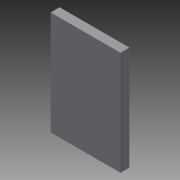
# Autodesk Inventor part: anker20Ah
Saved by Autodesk Inventor 2015 (Build 190159000, 159)
## iProperties
Created: 2014-09-23
Part Number: anker20Ah
Material: Generic
Document SubType Name: Modeling
Designer: ericd_000
Density: 1 g/cm^3
Appearance: Default
Author: ericd_000
Autodesk Inventor part; units mm, degrees
ref_plane "YZ Plane" through (0, 0, 0) normal (1, 0, 0) x (0, 1, 0)
ref_plane "XZ Plane" through (0, 0, 0) normal (0, 1, 0) x (-1, 0, 0)
ref_plane "XY Plane" through (0, 0, 0) normal (0, 0, 1) x (1, 0, 0)
sketch "Sketch1" plane through (0, 0, 0) normal (0, 1, 0) x (-1, 0, 0)
  line L0 (7.2949, 10.1037) -> (-117.7051, 10.1037)
  line L1 (-117.7051, 10.1037) -> (-117.7051, -175.8963)
  line L2 (-117.7051, -175.8963) -> (7.2949, -175.8963)
  line L3 (7.2949, -175.8963) -> (7.2949, 10.1037)
  point P0 (0, 0)
  dimension "d0" = 186
  dimension "d1" = 125
  constraints: 8 end point, 2 parallel, 1 horizontal, 1 perpendicular
  measures "d0" distance of L2.end L0.start
  measures "d1" distance of L0.start L0.end
extrude "Extrusion1" add sketch "Sketch1" along normal blind 16
body "Solid1"
